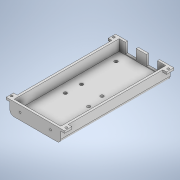
# Autodesk Inventor part: BOT_HOLDER_ENGR-2200
Saved by Autodesk Inventor 2022 (Build 260153000, 153)
## iProperties
Created: 2022-10-31
Part Number: BOT_HOLDER_ENGR-2200
Material: Generic
Document SubType Name: Modeling
Designer: udhay
Density: 1 g/cm^3
Appearance: Default
Author: udhay
## iProperties of the stored document BOT_HOLDER_ENGR-2200_3DPrint.ipt
Created: 2022-11-17
Part Number: BOT_HOLDER_ENGR-2200_3DPrint
Material: Generic
Document SubType Name: Modeling
Designer: udhay
Density: 1 g/cm^3
Appearance: Default
Author: udhay
Autodesk Inventor part; units mm, degrees
ref_plane "YZ Plane" through (0, 0, 0) normal (1, 0, 0) x (0, 1, 0)
ref_plane "XZ Plane" through (0, 0, 0) normal (0, 1, 0) x (-1, 0, 0)
ref_plane "XY Plane" through (0, 0, 0) normal (0, 0, 1) x (1, 0, 0)
sketch "Sketch7" plane through (0, 0, 0) normal (0, 0, 1) x (1, 0, 0)
  line L0 (0, 0) -> (70, 0)
  line L1 (70, 0) -> (70, 30)
  line L2 (70, 30) -> (0, 30)
  line L3 (0, 30) -> (0, 0)
  dimension "d25" = 70
  dimension "d26" = 30
  constraints: 8 end point, 2 parallel, 1 horizontal, 1 perpendicular
  measures "d25" distance of L2.end L1.end
  measures "d26" distance of L1.end L0.end
extrude "Extrusion5" add sketch "Sketch7" against normal blind 150
sketch "Sketch8" plane through (0, 30, 0) normal (0, 1, 0) x (1, 0, 0)
  line L0 (0, 0) -> (3, 0)
  line L1 (3, 0) -> (3, 3)
  line L2 (3, 3) -> (0, 3)
  line L3 (0, 3) -> (0, 0)
  line L4 (70, 150) -> (67, 150)
  line L5 (67, 150) -> (67, 147)
  line L6 (67, 147) -> (70, 147)
  line L7 (70, 147) -> (70, 150)
  line L8 (3, 3) -> (67, 3)
  line L9 (67, 3) -> (67, 147)
  line L10 (67, 147) -> (3, 147)
  line L11 (3, 147) -> (3, 3)
  dimension "d29" = 3
  dimension "d30" = 3
  dimension "d31" = 3
  dimension "d32" = 3
  constraints: 24 end point, 6 parallel, 3 horizontal, 3 perpendicular
  measures "d29" distance of L2.end L1.end
  measures "d30" distance of L1.end L0.end
  measures "d31" distance of L6.end L5.end
  measures "d32" distance of L5.end L4.end
extrude "Extrusion6" cut sketch "Sketch8" against normal blind 27 contours L11 L10 L9 L8
sketch "Sketch10" plane through (0, 0, -150) normal (0, 0, -1) x (-1, 0, 0)
  line L0 (-70, 30) -> (-70, 0) projected
  line L1 (-70, 0) -> (-61.5, 0)
  line L2 (-70, 4) -> (-70, 0)
  line L3 (0, 0) -> (0, 30) projected
  line L4 (0, 0) -> (-8.5, 0)
  line L5 (0, 4) -> (0, 0)
  line L6 (-54.5, 4) -> (-41.5, 4)
  line L7 (-61.5, 0) -> (-51.709, 0)
  line L8 (-8.5, 0) -> (-41.5, 0)
  line L9 (-26.0357, 0) -> (-23.5, 0)
  line L10 (-40.5, 4) -> (-40.5, 30)
  line L11 (-40.5, 30) -> (-55.5, 30)
  line L12 (-55.5, 30) -> (-55.5, 4)
  line L13 (-70, 0) -> (0, 0) projected
  line L14 (-55.5, 0) -> (-40.5, 0)
  line L15 (-55.5, 4) -> (-40.5, 4)
  line L16 (-11.5, 4) -> (-11.5, 30)
  line L17 (-11.5, 30) -> (-26.5, 30)
  line L18 (-26.5, 30) -> (-26.5, 4)
  line L19 (-26.5, 4) -> (-11.5, 4)
  point P0 (-48, 10)
  dimension "d188" = 15
  dimension "d189" = 15
  constraints: 34 end point, 5 horizontal, 2 parallel, 3 other
  measures "d188" distance of L11.end L10.end
  measures "d189" distance of L17.end L16.end
sketch "Sketch15" plane through (0, 0, -150) normal (0, 0, -1) x (-1, 0, 0)
  line L0 (-70, 30) -> (-70, 0) projected
  line L1 (0, 30) -> (0, 0) projected
  line L2 (-70, 30) -> (0, 30)
  line L3 (0, 30) -> (0, 18)
  line L4 (0, 18) -> (-70, 18)
  line L5 (-70, 18) -> (-70, 30)
  dimension "d100" = 12
  constraints: 8 end point, 2 parallel, 1 horizontal, 1 perpendicular, 1 point on line
  measures "d100" distance of L2.end L3.end
extrude "Extrusion10" cut sketch "Sketch15" against normal blind 10000
sketch "Sketch20" plane through (67, 3, -147) normal (-1, 0, 0) x (0, 0, 1)
  line L0 (0, 15) -> (144, 15)
  line L1 (144, 15) -> (144, 12)
  line L2 (144, 12) -> (0, 12)
  line L3 (0, 12) -> (0, 15)
  line L4 (0, 12) -> (2, 12)
  line L5 (2, 12) -> (2, 11)
  line L6 (2, 11) -> (0, 11)
  line L7 (0, 11) -> (0, 12)
  line L8 (144, 12) -> (142, 12)
  line L9 (142, 12) -> (142, 11)
  line L10 (142, 11) -> (144, 11)
  line L11 (144, 11) -> (144, 12)
  point P0 (147, -3)
  point P1 (2, 12)
  dimension "d132" = 144
  dimension "d133" = 3
  dimension "d134" = 2
  dimension "d135" = 1
  dimension "d136" = 2
  dimension "d137" = 1
  constraints: 24 end point, 6 parallel, 3 horizontal, 3 perpendicular
  measures "d132" distance of L1.end L2.end
  measures "d133" distance of L0.end L1.end
  measures "d134" distance of L5.end L6.end
  measures "d135" distance of L4.end L5.end
  measures "d136" distance of L10.end L9.end
  measures "d137" distance of L9.end L8.end
extrude "Extrusion17" cut sketch "Sketch20" against normal blind 1 contours L2 L5 L6 L7 | L11 L10 L9 L2
sketch "Sketch21" plane through (70, 0, 0) normal (1, 0, 0) x (0, 0, -1)
  line L0 (0, 0) -> (0, 18) projected
  line L1 (0, 18) -> (10, 18)
  line L2 (10, 18) -> (10, 15)
  line L3 (10, 15) -> (0, 15)
  line L4 (0, 15) -> (0, 18)
  line L5 (139.9948, 18) -> (149.9948, 18)
  line L6 (149.9948, 18) -> (149.9948, 15)
  line L7 (149.9948, 15) -> (139.9948, 15)
  line L8 (139.9948, 15) -> (139.9948, 18)
  dimension "d144" = 10
  dimension "d145" = 3
  dimension "d146" = 10
  dimension "d147" = 3
  constraints: 16 end point, 4 parallel, 2 horizontal, 2 perpendicular
  measures "d144" distance of L2.end L3.end
  measures "d145" distance of L1.end L2.end
  measures "d146" distance of L6.end L7.end
  measures "d147" distance of L5.end L6.end
extrude "Extrusion18" add sketch "Sketch21" along normal blind 5
sketch "Sketch23" plane through (0, 0, -150) normal (-1, 0, 0) x (0, 0, 1)
  line L0 (150, 18) -> (147, 18) projected
  line L1 (150, 18) -> (140, 18)
  line L2 (140, 18) -> (140, 15)
  line L3 (140, 15) -> (150, 15)
  line L4 (150, 15) -> (150, 18)
  line L5 (9.9944, 18) -> (-0.0056, 18)
  line L6 (-0.0056, 18) -> (-0.0056, 15)
  line L7 (-0.0056, 15) -> (9.9944, 15)
  line L8 (9.9944, 15) -> (9.9944, 18)
  point P0 (150, 0)
  point P1 (149.4, 18)
  point P2 (149.4, 18)
  dimension "d158" = 10
  dimension "d159" = 3
  dimension "d160" = 10
  dimension "d161" = 3
  constraints: 16 end point, 4 parallel, 2 horizontal, 2 perpendicular
  measures "d158" distance of L3.end L2.end
  measures "d159" distance of L2.end L1.end
  measures "d160" distance of L7.end L6.end
  measures "d161" distance of L6.end L5.end
extrude "Extrusion20" add sketch "Sketch23" along normal blind 5
sketch "Sketch25" plane through (3, 18, -147) normal (0, 1, 0) x (1, 0, 0)
  line L0 (72, -147) -> (-8, -147) projected
  line L1 (-8, -147) -> (-5.5, -147)
  line L2 (-8, -142) -> (-8, -147)
  line L3 (53.15, -147) -> (72, -147) projected
  line L4 (72, -147) -> (69.5, -147)
  line L5 (72, -142) -> (72, -147)
  line L6 (72, 2.9948) -> (69.5, 2.9948)
  line L7 (72, -2.0052) -> (72, 2.9948)
  line L8 (-8, 3.0056) -> (-8, -6.9944) projected
  line L9 (-8, 3.0056) -> (-5.5, 3.0056)
  line L10 (-8, -1.9944) -> (-8, 3.0056)
  circle A0 centre (-5.5, -1.9944) radius 1.5
  circle A1 centre (69.5, -2.0052) radius 1.5
  circle A2 centre (69.5, -142) radius 1.5
  circle A3 centre (-5.5, -142) radius 1.5
  point P0 (-3, -147)
  point P1 (10.85, -147)
  dimension "d180" = 3
  dimension "d181" = 3
  dimension "d182" = 3
  dimension "d183" = 3
  constraints: 16 end point, 4 centre point, 4 horizontal
  measures "d180" diameter of A0
  measures "d181" diameter of A1
  measures "d182" diameter of A2
  measures "d183" diameter of A3
extrude "Extrusion22" cut sketch "Sketch25" against normal blind 10
extrude "Extrusion23" cut sketch "Sketch10" against normal blind 10
sketch "Sketch26" plane through (0, 3, 0) normal (0, 1, 0) x (1, 0, 0)
  line L0 (3, 147) -> (67, 147) projected
  line L1 (3, 147) -> (13, 147)
  line L2 (3, 132.7) -> (3, 147)
  line L3 (61.5, 121.8573) -> (13, 121.8573)
  line L4 (16.5, 91.8787) -> (44.5, 91.8787)
  circle A0 centre (16.5, 81.9) radius 2.25
  circle A1 centre (44.5, 81.9) radius 2.25
  circle A2 centre (61.5, 132.7) radius 2.25
  circle A3 centre (13, 132.7) radius 2.25
  point P0 (0, 0)
  dimension "d195" = 48.5
  dimension "d200" = 28
  dimension "d233" = 4.5
  dimension "d234" = 4.5
  dimension "d235" = 4.5
  dimension "d236" = 4.5
  constraints: 8 end point, 4 centre point, 3 coincident, 1 horizontal
  measures "d195" distance of L3.start L3.end
  measures "d200" distance of L4.start L4.end
  measures "d233" diameter of A0
  measures "d234" diameter of A1
  measures "d235" diameter of A2
  measures "d236" diameter of A3
fillet "Face Fillet3" radius 5.5 1 edges at (70, 0, -75)
fillet "Face Fillet4" radius 5.5 1 edges at (0, 0, -75)
sketch "Sketch27" plane through (0, 0, 0) normal (0, 0, 1) x (1, 0, 0)
  line L0 (12.25, 28.2) -> (57.75, 28.2)
  line L1 (57.75, 28.2) -> (57.75, 7.8)
  line L2 (57.75, 7.8) -> (12.25, 7.8)
  line L3 (12.25, 7.8) -> (12.25, 28.2)
  line L4 (75, 18) -> (-5, 18) projected
  line L5 (57.75, 28.2) -> (12.25, 7.8) construction
  line L6 (12.25, 7.8) -> (12.75, 7.8)
  line L7 (12.25, 8.3) -> (12.25, 7.8)
  line L8 (57.75, 7.8) -> (57.25, 7.8)
  line L9 (57.75, 8.3) -> (57.75, 7.8)
  circle A0 centre (14.1, 9.65) radius 1.35
  line L10 (15.95, 7.8) -> (15.45, 7.8)
  circle A1 centre (55.9, 9.65) radius 1.35
  line L11 (57.75, 8.3) -> (57.75, 7.8)
  point P0 (0, 0)
  point P1 (35, 18)
  dimension "d210" = 45.5
  dimension "d211" = 20.4
  dimension "d218" = 2.7
  dimension "d219" = 0.5
  dimension "d221" = 2.7
  dimension "d223" = 0.5
  constraints: 22 end point, 3 horizontal, 2 centre point, 2 midpoint, 2 parallel, 1 perpendicular
  measures "d210" distance of L1.end L2.end
  measures "d211" distance of L0.end L1.end
  measures "d218" diameter of A0
  measures "d219" distance of L10.start L10.end
  measures "d221" diameter of A1
  measures "d223" distance of L11.start L11.end
extrude "Extrusion27" cut sketch "Sketch27" against normal blind 10 contours A0 | A1
sketch "Sketch28" plane through (0, 3, 0) normal (0, 1, 0) x (1, 0, 0)
  line L0 (51.8999, 76.8126) -> (11.6522, 76.8126)
  line L1 (11.6522, 76.8126) -> (11.6522, 60.3126)
  line L2 (51.8999, 60.3126) -> (51.8999, 76.8126)
  line L3 (51.8999, 58.2305) -> (51.8999, 60.3126)
  circle A0 centre (47.6999, 60.3126) radius 2.25
  line L4 (11.6522, 57.5365) -> (11.6522, 60.3126)
  circle A1 centre (15.8522, 60.3126) radius 2.25
  point P0 (0, 0)
  dimension "d226" = 16.5
  dimension "d228" = 4.5
  dimension "d230" = 4.5
  constraints: 10 end point, 2 centre point, 1 horizontal, 1 parallel, 1 perpendicular
  measures "d226" distance of L1.end L0.end
  measures "d228" diameter of A0
  measures "d230" diameter of A1
extrude "Extrusion28" cut sketch "Sketch28" against normal blind 10
extrude "Extrusion29" cut sketch "Sketch26" against normal blind 10
body "Solid3"
